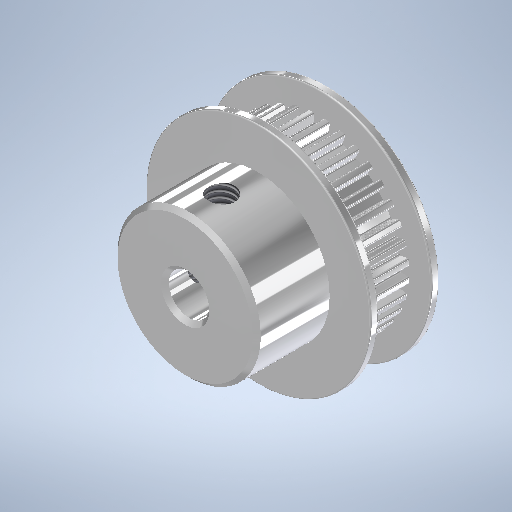
# Autodesk Inventor part: GT2_36T_5
Saved by Autodesk Inventor 2025.2 (Build 292293000, 293)
## iProperties
Created: 2014-01-09
Part Number: GT2_36T_5
Document SubType Name: Modeling
Designer: Matteo
Manufacturer: Standard
Standards Organization: Custom
Density: 1 g/cm^3
Material: Generic
Appearance: Aluminum - Flat
Author: Matteo
Autodesk Inventor part; units mm, degrees
ref_plane "YZ Plane" through (0, 0, 0) normal (1, 0, 0) x (0, 1, 0)
ref_plane "XZ Plane" through (0, 0, 0) normal (0, 1, 0) x (-1, 0, 0)
ref_plane "XY Plane" through (0, 0, 0) normal (0, 0, 1) x (1, 0, 0)
sketch "Schizzo1" plane through (0, 0, 0) normal (0, 0, 1) x (1, 0, 0)
  line L0 (-2.5, 0) -> (-8.85, 0)
  line L1 (-8.85, 0) -> (-8.85, 9)
  line L2 (-8.85, 9) -> (-13.9, 9)
  line L3 (-13.9, 9) -> (-13.9, 10)
  line L4 (-13.9, 10) -> (-11.2, 10)
  line L5 (-11.2, 10) -> (-11.2, 16.5)
  line L6 (-11.2, 16.5) -> (-13.9, 16.5)
  line L7 (-13.9, 16.5) -> (-13.9, 17.5)
  line L8 (-13.9, 17.5) -> (-2.5, 17.5)
  line L9 (-2.5, 17.5) -> (-2.5, 0)
  line L10 (0, 0) -> (0, 14.2963)
  point P0 (-13.9, 9.5)
  dimension "d0" = 5
  dimension "d1" = 17.7
  dimension "d2" = 27.8
  dimension "d3" = 1
  dimension "d4" = 6.5
  dimension "d5" = 17.5
  dimension "d6" = 22.4
  constraints: 22 end point, 5 horizontal, 2 vertical, 2 vertical alignment, 1 collinear, 1 horizontal alignment, 1 midpoint
  measures "d0" diameter of L9 L10
  measures "d1" diameter of L1 L10
  measures "d2" diameter of L7 L10
  measures "d3" distance of L6.end L7.end
  measures "d4" distance of L4.end L5.end
  measures "d5" distance of L8.end L0.start
  measures "d6" diameter of L5 L10
revolve "Rivoluzione1" add sketch "Schizzo1" angle 360 about axis through (0, 0, 0) along (0, 1, 0)
chamfer "Smusso1" distance 0.5 angle 45 1 edges at (8.85, 0, 0)
chamfer "Smusso2" distance 0.5 angle 45 2 edges at (2.5, 0, 0) (2.5, 17.5, 0)
sketch "Schizzo2" plane through (0, 0, 0) normal (1, 0, 0) x (0, 1, 0)
  line L0 (0, -8.35) -> (0, 8.35) projected
  line L1 (9, -13.9) -> (9, 13.9) projected
  line L2 (9, 0) -> (0, 0)
  point P0 (4.4907, -0.0034)
  constraints: 2 end point, 1 midpoint
hole "Foro1" at (0, 4.4907, -0.0034) direction (-1, 0, 0) diameter 3.242 end through all thread size "M4x0.7" class "6H" standard "ISO Metric profile"
pattern_circular "Serie circolare1" count 2 over 90 about axis through (0, 4.5, 0) along (0, 1, 0) of "Foro1"
sketch "Schizzo3" plane through (0, 16.5, 0) normal (0, -1, 0) x (1, 0, 0)
  circle A0 centre (0, 0) radius 13.9 projected
  line L0 (10.9744, 0.55) -> (10.2, 0.55)
  line L1 (10, 0.35) -> (10, -0.35)
  line L2 (10.2, -0.55) -> (10.9744, -0.55)
  circle A1 centre (0, 0) radius 11.2 projected
  arc A2 (10, -0.35) -> (10.2, -0.55) centre (10.2, -0.35) ccw
  arc A3 (10.2, 0.55) -> (10, 0.35) centre (10.2, 0.35) ccw
  circle A4 centre (0, 0) radius 13.9 projected
  circle A5 centre (0, 0) radius 3 projected
  arc A6 (11.1739, -0.7636) -> (11.1739, 0.7636) centre (0, 0) ccw
  arc A7 (11.1739, -0.7636) -> (10.9744, -0.55) centre (10.9744, -0.75) ccw
  arc A8 (10.9744, 0.55) -> (11.1739, 0.7636) centre (10.9744, 0.75) ccw
  point P0 (10, -0.55)
  point P1 (10, 0.55)
  point P2 (10, 0)
  dimension "d25" = 10
  dimension "d35" = 0.2
  dimension "d36" = 1.1
  dimension "d37" = 0.2
  constraints: 12 point on circle, 8 tangent, 6 end point, 5 centre point, 4 point on line, 2 equal radius, 2 horizontal, 1 coincident, 1 horizontal alignment, 1 midpoint
  measures "d25" distance from line of A0.centre L1
  measures "d35" radius of A2
  measures "d36" distance between parallel lines of L0 L2
  measures "d37" radius of A7
extrude "Estrusione1" cut sketch "Schizzo3" along normal up to surface (6.5 mm away) contours A8 A1 A7 L2 A2 L1 A3 L0 | A5 picked at (10.4, 0)
pattern_circular "Serie circolare2" count 36 over 360 about axis through (0, 13.25, 0) along (0, 1, 0) of "Estrusione1"
fillet "Raccordo4" radius 0.2 4 edges at (13.9, 9, 0) (13.9, 10, 0) (13.9, 16.5, 0) (13.9, 17.5, 0)
